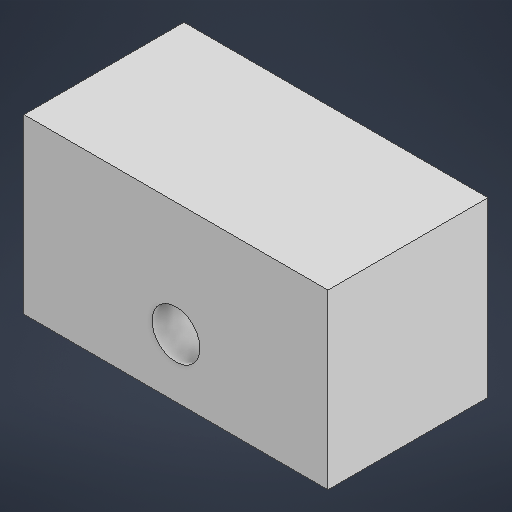
# Autodesk Inventor part: bruh
Saved by Autodesk Inventor 2026.2 (Build 302298000, 298)
## iProperties
Created: 2025-12-16
Part Number: bruh
Material: Generic
Document SubType Name: Modeling
Designer: Thoma
Density: 1 g/cm^3
Appearance: Default
Author: Thoma
Autodesk Inventor part; units mm, degrees
ref_plane "YZ Plane" through (0, 0, 0) normal (1, 0, 0) x (0, 1, 0)
ref_plane "XZ Plane" through (0, 0, 0) normal (0, 1, 0) x (-1, 0, 0)
ref_plane "XY Plane" through (0, 0, 0) normal (0, 0, 1) x (1, 0, 0)
sketch "Sketch1" plane through (0, 0, 0) normal (0, 0, 1) x (1, 0, 0)
  line L0 (-10, 11) -> (9, 11)
  line L1 (9, 11) -> (9, -10)
  line L2 (9, -10) -> (-10, -10)
  line L3 (-10, -10) -> (-10, 11)
  line L4 (-10, 0.8089) -> (9, 0.8089)
  point P0 (0, 0)
  constraints: 10 end point, 2 parallel, 2 perpendicular, 2 point on line, 1 horizontal
extrude "Extrusion1" add sketch "Sketch1" along normal blind 10 contours L4 L1 L2 L3
sketch "Sketch2" plane through (0, 0, 10) normal (0, 0, 1) x (1, 0, 0)
  line L0 (-10, -10) -> (9, -10) projected
  line L1 (-0.5, -10) -> (-0.5, -6.3365)
  circle A0 centre (-0.5, -6.3365) radius 1.5
  point P0 (0, 0)
  dimension "d2" = 3.6635
  dimension "d3" = 3
  constraints: 2 end point, 1 centre point, 1 coincident, 1 midpoint, 1 vertical
  measures "d2" distance of L1.start L1.end
  measures "d3" diameter of A0
extrude "Extrusion2" cut sketch "Sketch2" against normal blind 10
body "Solid1"
